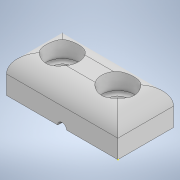
# Autodesk Inventor part: Top clamp for capillary jig - thermal seal
Saved by Autodesk Inventor 2020 (Build 240168000, 168)
## iProperties
Created: 2022-11-27
Part Number: Top clamp for capillary jig - thermal seal
Material: Generic
Document SubType Name: Modeling
Designer: Beaucage
Density: 1 g/cm^3
Appearance: Default
Author: Beaucage
Autodesk Inventor part; units mm, degrees
ref_plane "YZ Plane" through (0, 0, 0) normal (1, 0, 0) x (0, 1, 0)
ref_plane "XZ Plane" through (0, 0, 0) normal (0, 1, 0) x (-1, 0, 0)
ref_plane "XY Plane" through (0, 0, 0) normal (0, 0, 1) x (1, 0, 0)
sketch "Sketch1" plane through (0, 0, 0) normal (0, 1, 0) x (-1, 0, 0)
  line L0 (0, 0) -> (19.05, 0)
  line L1 (19.05, 0) -> (19.05, -9.525)
  line L2 (19.05, -9.525) -> (0, -9.525)
  line L3 (0, -9.525) -> (0, 0)
  dimension "d0" = 19.05
  dimension "d1" = 9.525
  constraints: 8 end point, 2 parallel, 1 horizontal, 1 perpendicular
  measures "d0" distance of L1.end L2.end
  measures "d1" distance of L0.end L1.end
extrude "Extrusion1" add sketch "Sketch1" along normal blind 6.35
sketch "Sketch2" plane through (-19.05, 0, 0) normal (0, 0, 1) x (1, 0, 0)
  line L0 (19.05, 0) -> (0, 0) projected
  point P0 (9.525, 0)
  constraints: 1 midpoint
hole "Hole1" at (-9.525, 0, 0) direction (0, 0, -1) diameter 1.5 end through all
sketch "Sketch3" plane through (0, 6.35, 0) normal (0, 1, 0) x (1, 0, 0)
  line L0 (-19.05, 0) -> (-10.275, 0) projected
  line L1 (-19.05, 0) -> (-14.2748, 0)
  line L2 (-14.2748, 0) -> (-14.2748, 4.7752)
  line L3 (-14.2748, 4.7752) -> (-19.05, 4.7752)
  line L4 (-19.05, 4.7752) -> (-19.05, 0)
  line L5 (-19.05, 0) -> (0, 0) projected
  line L6 (0, 0) -> (-4.7752, 0)
  line L7 (-4.7752, 0) -> (-4.7752, 4.7752)
  line L8 (-4.7752, 4.7752) -> (0, 4.7752)
  line L9 (0, 4.7752) -> (0, 0)
  dimension "d11" = 4.7752
  dimension "d12" = 4.7752
  dimension "d13" = 4.7752
  dimension "d14" = 4.7752
  constraints: 16 end point, 4 parallel, 2 horizontal, 2 perpendicular
  measures "d11" distance of L3.end L2.end
  measures "d12" distance of L2.end L1.end
  measures "d13" distance of L7.end L8.end
  measures "d14" distance of L6.end L7.end
hole "Hole2" at (-14.2748, 6.35, -4.7752) at (-4.7752, 6.35, -4.7752) direction (0, -1, 0) diameter 3.2766 end through all counterbore diameter 5.5626 counterbore depth 2.8448 clearance for "Socket Head Cap Screw" size "#4" standard "Ansi Unified Screw Threads"
sketch "Sketch4" plane through (0, 0, 0) normal (1, 0, 0) x (0, 0, -1)
  point P0 (0, 0)
fillet "Fillet1" radius 3.175 4 edges at (-9.525, 6.35, 0) (0, 6.35, -4.7625) (-9.525, 6.35, -9.525) (-19.05, 6.35, -4.7625)
body "Solid1"
